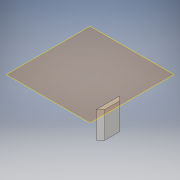
# Autodesk Inventor part: last_drill_slide_tolerance
Saved by Autodesk Inventor 2019 (Build 230136000, 136)
## iProperties
Created: 2018-12-20
Part Number: last_drill_slide_tolerance
Material: Generic
Document SubType Name: Modeling
Designer: assman
Density: 1 g/cm^3
Appearance: Default
Author: assman
## iProperties of the stored document last_drill_slide_tolerance_3DPrint.ipt
Created: 2018-12-20
Part Number: last_drill_slide_tolerance_3DPrint
Material: Generic
Document SubType Name: Modeling
Designer: assman
Density: 1 g/cm^3
Appearance: Default
Author: assman
Autodesk Inventor part; units mm, degrees
ref_plane "YZ Plane" through (0, 0, 0) normal (1, 0, 0) x (0, 1, 0)
ref_plane "XZ Plane" through (0, 0, 0) normal (0, 1, 0) x (-1, 0, 0)
ref_plane "XY Plane" through (0, 0, 0) normal (0, 0, 1) x (1, 0, 0)
ref_plane "Work Plane1" through (-10, 7, -20) normal (0, 1, 0) x (1, 0, 0)
sketch "Sketch3" plane through (-10, 7, -20) normal (0, 1, 0) x (1, 0, 0)
  line L0 (10, -5.9957) -> (8.5777, -7.418) projected
  line L1 (8.5777, -7.418) -> (8.5777, -0.6718) projected
  line L2 (8.5777, -0.6718) -> (10, -2.0942) projected
  line L3 (10, -5.9957) -> (10, -2.0942)
  line L4 (10, -5.9957) -> (8.5777, -7.418)
  line L5 (8.5777, -0.6718) -> (10, -2.0942)
  line L6 (8.5777, -7.418) -> (8.5777, -0.6718)
  line L7 (9.85, -2.1563) -> (9.85, -5.9336)
  line L8 (9.85, -5.9336) -> (8.7277, -7.0559)
  line L9 (8.7277, -7.0559) -> (8.7277, -1.034)
  line L10 (8.7277, -1.034) -> (9.85, -2.1563)
  point P0 (10, -20)
  dimension "d1" = 0.15
  constraints: 16 end point, 2 collinear, 2 perpendicular, 1 vertical, 3 other
  measures "d1" distance between parallel lines of L3 L7
extrude "Extrusion1" add sketch "Sketch3" against normal blind 7 contours L7 L8 L9 L10
body "Solid1"
